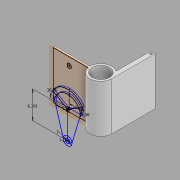
# Autodesk Inventor part: top_frame
Saved by Autodesk Inventor 2020 (Build 240168000, 168)
## iProperties
Created: 2020-03-09
Part Number: top_frame
Material: Generic
Document SubType Name: Modeling
Designer: xXxMrMayhemxXx
Density: 1 g/cm^3
Appearance: Default
Author: xXxMrMayhemxXx
Autodesk Inventor part; units mm, degrees
ref_plane "XZ Plane" through (0, 0, 0) normal (0, 1, 0) x (-1, 0, 0)
sketch "Sketch1" plane through (0, 0, 0) normal (0, 1, 0) x (-1, 0, 0)
  circle A0 centre (0, 0) radius 2
  circle A1 centre (0, 0) radius 2.5
  dimension "d0" = 4
  dimension "d1" = 5
  constraints: 2 centre point, 2 coincident
  measures "d0" diameter of A0
  measures "d1" diameter of A1
extrude "Extrusion1" add sketch "Sketch1" against normal blind 8
ref_plane "Work Plane2" through (0, 0, 0.5) normal (0, 0, 1) x (1, 0, 0)
sketch "Sketch3" plane through (0, 0, 0.5) normal (0, 0, 1) x (1, 0, 0)
  line L0 (-2.5, -8) -> (2.5, -8) projected
  line L1 (-2.5, 0) -> (-9.5, 0)
  line L2 (-10.5, -1) -> (-10.5, -7)
  line L3 (-9.5, -8) -> (-2.5, -8)
  line L4 (-2.5, -8) -> (-2.25, -8)
  line L5 (-2.25, -8) -> (-2.25, 0)
  line L6 (2.5, 0) -> (-2.5, 0) projected
  line L7 (-2.25, 0) -> (-2.5, 0)
  line L8 (-9.5, -8) -> (-10.5, -8)
  line L9 (-10.5, -8) -> (-10.5, -7)
  line L10 (-9.5, 0) -> (-10.5, 0)
  line L11 (-10.5, -1) -> (-10.5, 0)
  point P0 (0, 0)
  point P1 (-9.5, -1)
  dimension "d6" = 8
  dimension "d8" = 0.25
  constraints: 20 end point, 3 point on line, 2 collinear, 2 horizontal, 2 parallel, 2 perpendicular
  measures "d6" distance of L1.start L10.end
  measures "d8" distance of L3.end L4.end
extrude "Extrusion2" add sketch "Sketch3" against normal blind 0.5
sketch "Sketch13" plane through (0, 0, 0.5) normal (0, 0, 1) x (1, 0, 0)
  circle A0 centre (-6.8, -7.25) radius 0.25
  line L0 (-2.4495, 0) -> (-2.4495, -8) projected
  line L1 (-2.4495, 0) -> (-10.5, 0) projected
  line L2 (-10.5, 0) -> (-10.5, -8) projected
  line L3 (-10.5, -8) -> (-2.4495, -8) projected
  point P0 (0, 0)
  dimension "d77" = 0.5
  dimension "d78" = 3.7
  dimension "d79" = 0.75
  constraints: 1 centre point
  measures "d77" diameter of A0
  measures "d78" distance from line of L2 A0.centre
  measures "d79" distance from line of L3 A0.centre
extrude "Extrusion12" cut sketch "Sketch13" against normal through all contours A0
ref_plane "Work Plane3" through (2, 0, 0) normal (1, 0, 0) x (0, 1, 0)
sketch "Sketch16" plane through (2, 0, 0) normal (1, 0, 0) x (0, 1, 0)
  line L0 (-8, 0) -> (-8, 0.5) projected
  line L1 (-8, 0) -> (-8, -10)
  line L2 (-8, -10) -> (0, -10)
  line L3 (0, -10) -> (0, 0)
  line L4 (-8, 0) -> (0, 0) projected
  dimension "d63" = 10
  constraints: 6 end point, 2 parallel, 2 perpendicular
  measures "d63" distance between parallel lines of L2 L4
extrude "Extrusion15" add sketch "Sketch16" along normal mid plane 1
sketch "Sketch17" plane through (0, 0, 0) normal (0, 1, 0) x (1, 0, 0)
  circle A0 centre (0, 0) radius 2
  circle A1 centre (0, 0) radius 2.5
  line L0 (1.5, 0) -> (1.5, 1.3229) projected
  line L1 (1.5, 0) -> (2, 0) projected
  line L2 (2.5, 10) -> (2.5, 0) projected
  dimension "d67" = 5
  dimension "d66" = 4
  constraints: 2 coincident, 1 centre point, 1 horizontal alignment, 1 other
  measures "d66" diameter of A0
extrude "Extrusion16" cut sketch "Sketch17" against normal through all contours L1 L0 A0 picked at (1.5908, 0.7499)
sketch "Sketch18" plane through (0, -8, 0) normal (0, -1, 0) x (1, 0, 0)
  line L0 (1.5, -10) -> (2.5, -10) projected
  line L1 (2.5, 0) -> (2.5, -10) projected
  line L2 (1.5, -10) -> (1.5, -2) projected
  line L3 (1.5, -9.5) -> (2.5, -9.5)
  line L4 (2, -10) -> (2, -9.5)
  circle A0 centre (2, -9.5) radius 0.25
  point P0 (0, 0)
  dimension "d70" = 0.5
  dimension "d71" = 0.5
  constraints: 4 end point, 2 midpoint, 2 point on line, 1 centre point, 1 coincident, 1 horizontal, 1 parallel
  measures "d70" diameter of A0
  measures "d71" distance of L4.start L4.end
extrude "Extrusion17" cut sketch "Sketch18" against normal through all contours A0 L3 L4 | L4 L3 A0 | A0 L3
sketch "Sketch19" plane through (0, 0, 0) normal (0, 1, 0) x (1, 0, 0)
  circle A0 centre (2, 9.5) radius 0.25 projected
  circle A1 centre (0, 0) radius 2 projected
  arc A2 (1.5, 2) -> (-2.5, 0) centre (0, 0) ccw projected
  line L0 (-10.5, 0) -> (-2.5, 0) projected
  line L1 (-10.5, -0.5) -> (-10.5, 0) projected
  line L2 (-2.4495, -0.5) -> (-10.5, -0.5) projected
  arc A3 (-2.4495, -0.5) -> (2.5, 0) centre (0, 0) ccw projected
  line L3 (2.5, 10) -> (2.5, 0) projected
  line L4 (1.5, 10) -> (2.5, 10) projected
  line L5 (1.5, 2) -> (1.5, 10) projected
extrude "Extrusion18" add sketch "Sketch19" along normal blind 3
sketch "Sketch20" plane through (0, 0, 0.5) normal (0, 0, 1) x (1, 0, 0)
  circle A0 centre (-6.8, -7.25) radius 0.25 projected
  circle A1 centre (-6.8, -7.25) radius 0.25 projected
  circle A2 centre (-6.8, 1.199) radius 0.5
  point P0 (0, 0)
  dimension "d82" = 1
  dimension "d83" = 8.449
  constraints: 1 centre point
  measures "d82" diameter of A2
  measures "d83" distance of A2.centre A0.centre
extrude "Extrusion19" cut sketch "Sketch20" against normal through all contours A2
sketch "Sketch21" plane through (0, 0, 0.5) normal (0, 0, 1) x (1, 0, 0)
  circle A0 centre (-6.8, -7.25) radius 0.25 projected
  circle A1 centre (-6.8, 1.199) radius 0.5 projected
  circle A2 centre (-6.8, -7.25) radius 0.25 projected
  line L0 (-2.4495, 3) -> (-2.4495, -8) projected
  line L1 (-10.5, 3) -> (-2.4495, 3) projected
  line L2 (-10.5, 3) -> (-10.5, -8) projected
  line L3 (-10.5, -8) -> (-2.4495, -8) projected
  line L4 (-6.8, -7.25) -> (-9.8, -7.25)
  line L5 (-6.8, -7.25) -> (-3.8, -7.25)
  arc A3 (-3.8, -7.25) -> (-9.8, -7.25) centre (-6.8, -7.25) ccw
  arc A4 (-3.3359, -5.25) -> (-10.2641, -5.25) centre (-6.8, -7.25) ccw
  line L6 (-6.8, -7.25) -> (-3.3359, -5.25)
  line L7 (-6.8, -7.25) -> (-10.2641, -5.25)
  point P0 (0, 0)
  dimension "d86" = 3
  dimension "d87" = 3
  dimension "d92" = 3
  dimension "d93" = 1
  dimension "d94" = 30
  dimension "d95" = 30
  constraints: 8 end point, 4 point on circle, 2 centre point, 1 horizontal, 1 point on line
  measures "d86" distance of L4.start L4.end
  measures "d87" distance of L4.start L5.end
  measures "d92" radius of A3
  measures "d93" radial gap between concentric circles of A3 A4
  measures "d94" angle of L5 L6
  measures "d95" angle of L7 L4
ref_plane "Work Plane4" through (0, 0, 0.9) normal (0, 0, 1) x (1, 0, 0)
sketch "Sketch22" plane through (0, 0, 0.9) normal (0, 0, 1) x (1, 0, 0)
  arc A0 (-3.3359, -5.25) -> (-10.2641, -5.25) centre (-6.8, -7.25) ccw projected
  arc A1 (-3.8, -7.25) -> (-9.8, -7.25) centre (-6.8, -7.25) ccw projected
  line L0 (-6.8, -7.25) -> (-3.3359, -5.25) projected
  line L1 (-6.8, -7.25) -> (-10.2641, -5.25) projected
  circle A2 centre (-6.8, -7.25) radius 0.25 projected
  circle A3 centre (-6.8, -7.25) radius 0.25 projected
  line L2 (-6.8, -7.25) -> (-6.8, -13.551)
  circle A4 centre (-6.8, -13.551) radius 0.5
  circle A5 centre (-6.8, -13.551) radius 1
  line L3 (-6.8, -13.551) -> (-5.8, -13.551)
  line L4 (-6.8, -13.551) -> (-7.8, -13.551)
  line L5 (-5.8, -13.551) -> (-3.3359, -5.25)
  line L6 (-7.8, -13.551) -> (-10.2641, -5.25)
  point P0 (0, 0)
  dimension "d97" = 1
  dimension "d98" = 6.301
  dimension "d99" = 2
  constraints: 10 end point, 2 centre point, 2 coincident, 2 point on circle, 1 perpendicular, 1 point on line, 1 vertical
  measures "d97" diameter of A4
  measures "d98" distance of L2.start L2.end
  measures "d99" diameter of A5
body "Solid1"
